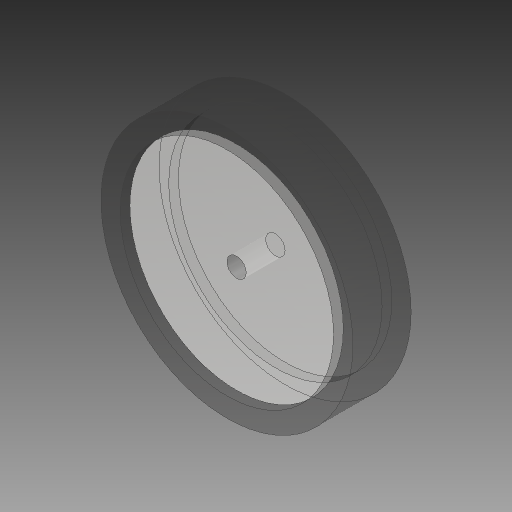
# Autodesk Inventor part: Koło
Saved by Autodesk Inventor 2018 (Build 220112000, 112)
## iProperties
Created: 2018-08-11
Part Number: Koło
Material: Tworzywo sztuczne PET
Document SubType Name: Modeling
Designer: Wojciech
Density: 1.541 g/cm^3
Appearance: Poliwęglan — przezroczysty
Mass: 58.0943 g
Surface Area: 106.814 cm^2
Volume: 37.6991 cm^3
Author: Wojciech
Autodesk Inventor part; units mm, degrees
ref_plane "YZ Plane" through (0, 0, 0) normal (1, 0, 0) x (0, 1, 0)
ref_plane "XZ Plane" through (0, 0, 0) normal (0, 1, 0) x (-1, 0, 0)
ref_plane "XY Plane" through (0, 0, 0) normal (0, 0, 1) x (1, 0, 0)
sketch "Szkic1" plane through (0, 0, 0) normal (0, 0, 1) x (1, 0, 0)
  circle A0 centre (0, 0) radius 27.5
  dimension "d0" = 55
  constraints: 1 centre point, 1 coincident
  measures "d0" diameter of A0
extrude "Wyciągnięcie proste1" add sketch "Szkic1" along normal mid plane 10
sketch "Szkic3" plane through (0, 0, 0) normal (0, 0, 1) x (1, 0, 0)
  circle A0 centre (0, 0) radius 32.5
  circle A1 centre (0, 0) radius 27.5
  dimension "d4" = 65
  dimension "d5" = 55
  constraints: 2 centre point, 2 coincident
  measures "d4" diameter of A0
  measures "d5" diameter of A1
extrude "Wyciągnięcie proste2" add sketch "Szkic3" along normal mid plane 15
sketch "Szkic4" plane through (0, 0, -7.5) normal (0, 0, -1) x (-1, 0, 0)
  point P0 (0, 0)
  point P1 (0, 0)
  constraints: 1 coincident
hole "Otwór1" at (0, 0, -7.5) direction (0, 0, 1) diameter 5 end through all
